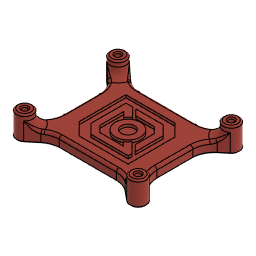
Toolhead Breakout PCB Mount (Autodesk Fusion 360 design; units mm, degrees)
Autodesk Fusion 360 part; units mm, degrees
sketch "Sketch1" plane through (0, 0, 0) normal (0, 0, 1) x (1, 0, 0)
  line L0 (21.185, 17.41) -> (-21.185, 17.41) construction
  line L1 (-21.185, 17.41) -> (-21.185, -17.41) construction
  line L2 (-21.185, -17.41) -> (21.185, -17.41) construction
  line L3 (21.185, -17.41) -> (21.185, 17.41) construction
  line L4 (21.185, 17.41) -> (-21.185, -17.41) construction
  line L5 (-21.185, 17.41) -> (21.185, -17.41) construction
  circle A0 centre (-21.185, 17.41) radius 0.95
  circle A1 centre (-21.185, -17.41) radius 0.95
  circle A2 centre (21.185, -17.41) radius 0.95
  circle A3 centre (21.185, 17.41) radius 0.95
  circle A4 centre (-21.185, 17.41) radius 3
  line L6 (-23.089743, 15.092253) -> (-17.5, 10.498558)
  line L7 (17.5, 15) -> (-17.5, 15)
  line L8 (-17.5, 15) -> (-17.5, -15)
  line L9 (-17.5, -15) -> (17.5, -15)
  line L10 (17.5, -15) -> (17.5, 15)
  line L11 (17.5, 15) -> (-17.5, -15) construction
  line L12 (-17.5, 15) -> (17.5, -15) construction
  line L13 (-13.527395, 15) -> (-19.280257, 19.727747)
  circle A5 centre (21.185, 17.41) radius 3
  circle A6 centre (21.185, -17.41) radius 3
  circle A7 centre (-21.185, -17.41) radius 3
  line L14 (0, 0) -> (0, 14.463533) construction
  line L15 (0, 0) -> (27.885284, 0) construction
  line L16 (23.089743, 15.092253) -> (17.5, 10.498558)
  line L17 (13.527395, 15) -> (19.280257, 19.727747)
  line L18 (-23.089743, -15.092253) -> (-17.5, -10.498558)
  line L19 (-13.527395, -15) -> (-19.280257, -19.727747)
  line L20 (13.527395, -15) -> (19.280257, -19.727747)
  line L21 (23.089743, -15.092253) -> (17.5, -10.498558)
  dimension "d1" = 42.37
  dimension "d2" = 34.82
  dimension "d3" = 1.9
  dimension "d4" = 6
  dimension "d5" = 35
  dimension "d6" = 30
  constraint horizontal L0
  constraint perpendicular L0 L1
  constraint parallel L0 L2
  constraint parallel L1 L3
  constraint coincident L4 L14.start
  constraint coincident L5 L14.start
  constraint coincident L14.start L15.start
  constraint coincident L0.end L1.start
  constraint coincident L1.end L2.start
  constraint coincident L2.end L3.start
  constraint coincident L0.start L3.end
  constraint equal A0 A3
  constraint equal A0 A1
  constraint equal A0 A2
  constraint concentric A0 A4
  constraint parallel L5 L6
  constraint tangent A4 L6
  constraint horizontal L7
  constraint perpendicular L7 L8
  constraint parallel L7 L9
  constraint parallel L8 L10
  constraint coincident L11 L14.start
  constraint coincident L12 L14.start
  constraint parallel L6 L13
  constraint tangent A4 L13
  constraint concentric A3 A5
  constraint concentric A2 A6
  constraint concentric A1 A7
  constraint equal A4 A5
  constraint equal A4 A7
  constraint equal A4 A6
  constraint perpendicular L0 L14
  constraint perpendicular L14 L15
  measures "d1" distance of L0.start L0.end
  measures "d2" distance of L0.end L1.end
  measures "d3" diameter of A3
  measures "d4" diameter of A4
  measures "d5" distance of L8.end L9.end
  measures "d6" distance of L7.start L9.end
extrude "Extrude1" add sketch "Sketch1" along normal blind 4 contours A4 | A4 L6 L7 L8 L13 | L7 L8 L9 L10 | L7 L10 A5 L16 L17 | L8 L9 A7 L18 L19 | A5 | A7 | L9 L10 A6 L20 L21 | A6 picked at (-23.211986, 16.300895) picked at (-18.178122, 13.467827) picked at (-4.509132, 5) picked at (18.241117, 13.429571) picked at (-18.178122, -13.467827) picked at (20.230473, 15.305799) picked at (-23.492473, -17.290207) picked at (18.241117, -13.429571) picked at (19.574982, -19.067295)
extrude "Extrude4" add sketch "Sketch1" along normal blind 9 contours A4 | A5 | A7 | A6 picked at (-23.211986, 16.300895) picked at (20.230473, 15.305799) picked at (-23.492473, -17.290207) picked at (19.574982, -19.067295)
fillet "Fillet1" radius 8 8 edges at (-17.5, 10.498558, 2) (-17.5, -10.498558, 2) (13.527395, -15, 2) (-13.527395, -15, 2) (17.5, 10.498558, 2) (17.5, -10.498558, 2) (-13.527395, 15, 2) (13.527395, 15, 2)
fillet "Fillet2" radius 3 4 edges at (-18.867253, -15.505257, 4) (-18.867253, 15.505257, 4) (18.867253, 15.505257, 4) (18.867253, -15.505257, 4)
fillet "Fillet3" radius 1 28 edges at (17.673949, 18.407671, 5.136394) (15.498674, 16.627726, 4.011298) (13.073986, 15.372296, 4) (0, 15, 4) (-13.073986, 15.372296, 4) (-15.493793, 16.624024, 4.010844) (-17.673949, 18.407671, 5.136394) (-21.842955, 14.067632, 5.492495) (-19.869307, 12.400515, 4.114665) (-17.953285, 9.372776, 4) (-17.5, 0, 4) (-17.953285, -9.372776, 4) (-19.767407, -12.298339, 4.081732) (-21.842955, -14.067632, 5.492495) (-17.673949, -18.407671, 5.136394) (-15.512805, -16.638953, 4.012567) (-13.073986, -15.372296, 4) (0, -15, 4) (13.073986, -15.372296, 4) (15.511912, -16.637827, 4.01259) (17.673949, -18.407671, 5.136394) (21.842955, -14.067632, 5.492495) (19.869307, -12.400515, 4.114665) (17.953285, -9.372776, 4) (17.5, 0, 4) (17.953285, 9.372776, 4) (19.767407, 12.298339, 4.081732) (21.842955, 14.067632, 5.492495)
chamfer "Chamfer1" distance 0.4 angle 45 4 edges at (20.299289, -17.066465, 9) (20.299289, 17.753535, 9) (-22.070711, 17.753535, 9) (-22.070711, -17.066465, 9)
fillet "Fillet4" radius 0.6 4 edges at (18.388018, -18.494846, 9) (18.388018, 16.325154, 9) (-23.981982, 16.325154, 9) (-23.981982, -18.494846, 9)
sketch "Sketch5" plane through (0, 0, 4) normal (0, 0, 1) x (-1, 0, 0)
  arc A0 (-18.316523, -12.1401) -> (-16.5, -6.718139) centre (-25.5, -6.718139) ccw
  arc A1 (-15.522684, -15.425514) -> (-18.316523, -12.1401) centre (-21.185, -17.41) ccw
  arc A2 (-10.661906, -14) -> (-15.522684, -15.425514) centre (-10.661906, -23) ccw
  line L0 (-10.661906, -14) -> (10.661906, -14)
  arc A3 (15.522684, -15.425514) -> (10.661906, -14) centre (10.661906, -23) ccw
  arc A4 (18.316523, -12.1401) -> (15.522684, -15.425514) centre (21.185, -17.41) ccw
  arc A5 (16.5, -6.718139) -> (18.316523, -12.1401) centre (25.5, -6.718139) ccw
  line L1 (16.5, -6.718139) -> (16.5, 6.718139)
  arc A6 (18.316523, 12.1401) -> (16.5, 6.718139) centre (25.5, 6.718139) ccw
  arc A7 (15.522684, 15.425514) -> (18.316523, 12.1401) centre (21.185, 17.41) ccw
  arc A8 (10.661906, 14) -> (15.522684, 15.425514) centre (10.661906, 23) ccw
  line L2 (10.661906, 14) -> (-10.661906, 14)
  arc A9 (-15.522684, 15.425514) -> (-10.661906, 14) centre (-10.661906, 23) ccw
  arc A10 (-18.316523, 12.1401) -> (-15.522684, 15.425514) centre (-21.185, 17.41) ccw
  arc A11 (-16.5, 6.718139) -> (-18.316523, 12.1401) centre (-25.5, 6.718139) ccw
  line L3 (-16.5, 6.718139) -> (-16.5, -6.718139)
  line L4 (3.041112, -4.747588) -> (6.380937, -8.147472)
  line L5 (5.407317, 8.457348) -> (-8.557371, 8.457348)
  line L6 (8.951193, -8.147472) -> (8.951193, 4.858068)
  line L7 (4.356513, 6.20562) -> (6.617025, 3.89712)
  arc A12 (-4.696496, 3.159381) -> (-3.040035, 4.808515) centre (0.041673, 0.05664) cw
  line L8 (-8.557263, 5.8872) -> (-8.557263, -4.545672)
  line L9 (-8.557263, -4.545672) -> (-5.026275, -8.138112)
  line L10 (-8.557371, 7.088376) -> (-4.696496, 3.159381)
  line L11 (-6.221367, 3.506448) -> (-8.557263, 5.8872)
  line L12 (11.678625, -10.865292) -> (-6.698583, -10.866948)
  line L13 (11.678301, 6.510792) -> (11.678625, -10.865292)
  line L14 (7.093197, 11.18478) -> (11.678301, 6.510792)
  line L15 (6.617025, 3.89712) -> (6.630262, -5.068835)
  line L16 (-11.180835, -6.308232) -> (-11.180835, 11.184456)
  line L17 (2.992077, -5.888004) -> (-3.966219, -5.888004)
  line L18 (-11.180835, 11.184456) -> (7.093197, 11.18478)
  line L19 (-3.040035, 4.808515) -> (-4.420074, 6.20562)
  arc A13 (4.717839, -3.13878) -> (3.041112, -4.747588) centre (0.041673, 0.05664) cw
  line L20 (-4.420074, 6.20562) -> (4.356513, 6.20562)
  line L21 (-6.221367, -3.586668) -> (-6.221367, 3.506448)
  line L22 (8.951193, 4.858068) -> (5.407317, 8.457348)
  line L23 (6.380937, -8.147472) -> (8.951193, -8.147472)
  circle A14 centre (0.004302, 0.020115) radius 4.75128
  line L24 (-5.026275, -8.138112) -> (5.217201, -8.138112)
  line L25 (6.630262, -5.068835) -> (4.717839, -3.13878)
  line L26 (-8.557371, 8.457348) -> (-8.557371, 7.088376)
  line L27 (-6.698583, -10.866948) -> (-11.180835, -6.308232)
  line L28 (-3.966219, -5.888004) -> (-6.221367, -3.586668)
  circle A15 centre (0.004302, 0.020115) radius 2.499624
  line L29 (5.217201, -8.138112) -> (2.992077, -5.888004)
extrude "Extrude6" cut sketch "Sketch5" against normal blind 1 contours L12 L13 L14 L16 L18 L27 | A15 picked at (3.399081, -9.956784) picked at (-0.309409, 0.671543)
chamfer "Chamfer2" distance 0.4 angle 45 1 faces at (3.553969, -5, 0)
